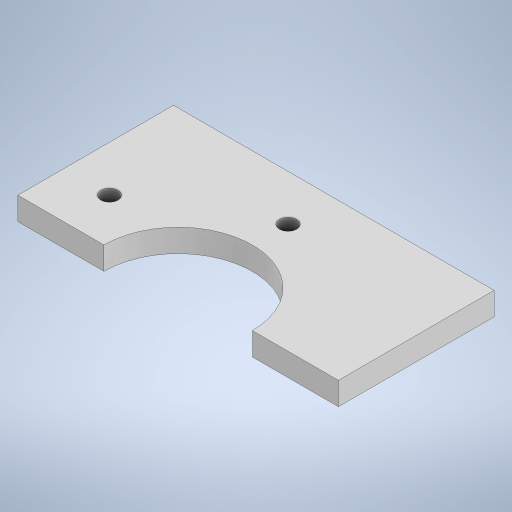
# Autodesk Inventor part: InventorPart1Commit3
Saved by Autodesk Inventor 2023 (Build 270158000, 158)
## iProperties
Created: 2023-03-15
Part Number: InventorPart1Commit3
Material: Generic
Document SubType Name: Modeling
Designer: ianjo
Density: 1 g/cm^3
Appearance: Default
Author: ianjo
Autodesk Inventor part; units mm, degrees
ref_plane "YZ Plane" through (0, 0, 0) normal (1, 0, 0) x (0, 1, 0)
ref_plane "XZ Plane" through (0, 0, 0) normal (0, 1, 0) x (-1, 0, 0)
ref_plane "XY Plane" through (0, 0, 0) normal (0, 0, 1) x (1, 0, 0)
sketch "Sketch1" plane through (0, 0, 0) normal (0, 1, 0) x (-1, 0, 0)
  line L0 (43.4289, -18.5999) -> (-45.4711, -18.5999)
  line L1 (-45.4711, -18.5999) -> (-45.4711, 24.5801)
  line L2 (-45.4711, 24.5801) -> (43.4289, 24.5801)
  line L3 (43.4289, 24.5801) -> (43.4289, -18.5999)
  point P0 (0, 0)
  dimension "d2" = 88.9
  dimension "d3" = 43.18
  constraints: 8 end point, 2 parallel, 1 horizontal, 1 perpendicular
  measures "d2" distance of L1.end L2.end
  measures "d3" distance of L0.end L1.end
extrude "Extrusion1" add sketch "Sketch1" along normal blind 6.35
sketch "Sketch2" plane through (0, 6.35, 0) normal (0, 1, 0) x (1, 0, 0)
  line L0 (45.4711, -24.5801) -> (45.4711, 18.5999) projected
  line L1 (45.4711, 18.5999) -> (-43.4289, 18.5999) projected
  point P0 (0, 0)
  point P1 (1.0211, -24.5835)
  dimension "d22" = 44.45
  dimension "d23" = 43.1834
  measures "d22" distance from line of L0 point (1.021, -24.583)
  measures "d23" distance from line of L1 point (1.021, -24.583)
hole "Hole1" at (1.0211, 6.35, 24.5835) direction (0, -1, 0) diameter 41.148 end through all
sketch "Sketch3" plane through (0, 6.35, 0) normal (0, 1, 0) x (1, 0, 0)
  line L0 (-43.4289, 18.5999) -> (-43.4289, -24.5801) projected
  line L1 (-43.4289, -24.5801) -> (-19.5529, -24.5801) projected
  point P0 (0, 0)
  point P1 (-30.7289, -11.8801)
  dimension "d13" = 12.7
  dimension "d14" = 12.7
  measures "d13" distance from line of L0 point (-30.729, -11.88)
  measures "d14" distance from line of L1 point (-30.729, -11.88)
hole "Hole2" at (-30.7289, 6.35, 11.8801) direction (0, -1, 0) diameter 4.826 end through all
sketch "Sketch4" plane through (0, 6.35, 0) normal (0, 1, 0) x (1, 0, 0)
  line L0 (45.4711, 18.5999) -> (-43.4289, 18.5999) projected
  line L1 (45.4711, -24.5801) -> (45.4711, 18.5999) projected
  point P0 (0, 0)
  point P1 (1.0211, 5.8999)
  dimension "d24" = 12.7
  dimension "d25" = 44.45
  measures "d24" distance from line of L0 point (1.021, 5.9)
  measures "d25" distance from line of L1 point (1.021, 5.9)
hole "Hole3" at (1.0211, 6.35, -5.8999) direction (0, -1, 0) diameter 4.826 end through all
body "Solid1"
